Autodesk Fusion 360 part; units mm, degrees
(part 8 of 25)
sketch "Botton Trace" plane through (0, 0, 0) normal (0, 0, 1) x (1, 0, 0)
  arc A0 (82.7578, 33.1788) -> (82.7578, 32.8613) centre (82.7578, 33.0201) ccw
  arc A1 (15.6337, 33.8137) -> (15.6337, 33.4963) centre (15.6337, 33.655) ccw
  arc A2 (82.4468, 33.8137) -> (82.4468, 33.4963) centre (82.4468, 33.655) ccw
  arc A3 (66.04, 33.1788) -> (66.04, 32.8613) centre (66.04, 33.0201) ccw
  arc A4 (81.28, 32.8613) -> (81.28, 33.1788) centre (81.28, 33.0201) ccw
  arc A5 (66.04, 33.4963) -> (66.04, 33.8137) centre (66.04, 33.655) ccw
  arc A6 (0.7747, 33.8137) -> (0.7747, 33.4963) centre (0.7747, 33.655) ccw
  arc A7 (52.818, 33.8137) -> (52.818, 33.4963) centre (52.818, 33.655) ccw
  arc A8 (15.7861, 33.4963) -> (15.7861, 33.8137) centre (15.7861, 33.655) ccw
  arc A9 (71.8947, 32.8613) -> (71.8947, 33.1788) centre (71.8947, 33.0201) ccw
  arc A10 (81.28, 33.8137) -> (81.28, 33.4963) centre (81.28, 33.655) ccw
  arc A11 (35.9156, 33.8137) -> (35.9156, 33.4963) centre (35.9156, 33.655) ccw
  arc A12 (39.1736, 33.4963) -> (39.1736, 33.8137) centre (39.1736, 33.655) ccw
  arc A13 (11.289, 33.8137) -> (11.289, 33.4963) centre (11.289, 33.655) ccw
  arc A14 (52.2859, 33.1788) -> (52.2859, 32.8613) centre (52.2859, 33.0201) ccw
  arc A15 (33.2611, 32.8613) -> (33.2611, 33.1788) centre (33.2611, 33.0201) ccw
  arc A16 (84.2253, 32.8613) -> (84.2253, 33.1788) centre (84.2253, 33.0201) ccw
  arc A17 (17.7419, 33.8137) -> (17.7419, 33.4963) centre (17.7419, 33.655) ccw
  arc A18 (35.3189, 33.1788) -> (35.3189, 32.8613) centre (35.3189, 33.0201) ccw
  arc A19 (31.002, 33.4963) -> (31.002, 33.8137) centre (31.002, 33.655) ccw
  arc A20 (48.6064, 33.1788) -> (48.6064, 32.8613) centre (48.6064, 33.0201) ccw
  arc A21 (17.7419, 33.1788) -> (17.7419, 32.8613) centre (17.7419, 33.0201) ccw
  arc A22 (49.3141, 32.8613) -> (49.3141, 33.1788) centre (49.3141, 33.0201) ccw
  arc A23 (54.9021, 32.8613) -> (54.9021, 33.1788) centre (54.9021, 33.0201) ccw
  arc A24 (84.2253, 33.4963) -> (84.2253, 33.8137) centre (84.2253, 33.655) ccw
  arc A25 (28.2956, 34.4487) -> (28.2956, 34.1313) centre (28.2956, 34.29) ccw
  arc A26 (0.7747, 35.0838) -> (0.7747, 34.7663) centre (0.7747, 34.925) ccw
  line L0 (61.7097, 34.29) -> (62.7503, 34.29)
  arc A27 (84.2253, 34.1313) -> (84.2253, 34.4487) centre (84.2253, 34.29) ccw
  arc A28 (72.517, 34.1313) -> (72.517, 34.4487) centre (72.517, 34.29) ccw
  arc A29 (61.7097, 34.4487) -> (61.7097, 34.1313) centre (61.7097, 34.29) ccw
  arc A30 (17.7419, 34.4487) -> (17.7419, 34.1313) centre (17.7419, 34.29) ccw
  arc A31 (79.7179, 34.4487) -> (79.7179, 34.1313) centre (79.7179, 34.29) ccw
  arc A32 (25.0444, 34.1313) -> (25.0444, 34.4487) centre (25.0444, 34.29) ccw
  arc A33 (56.974, 35.0838) -> (56.974, 34.7663) centre (56.974, 34.925) ccw
  arc A34 (57.1337, 34.4487) -> (57.1337, 34.1313) centre (57.1337, 34.29) ccw
  arc A35 (12.6332, 34.7663) -> (12.6332, 35.0838) centre (12.6332, 34.925) ccw
  arc A36 (60.2103, 34.1313) -> (60.2103, 34.4487) centre (60.2103, 34.29) ccw
  arc A37 (15.613, 34.4487) -> (15.613, 34.1313) centre (15.613, 34.29) ccw
  arc A38 (30.367, 34.1313) -> (30.367, 34.4487) centre (30.367, 34.29) ccw
  arc A39 (54.6263, 34.1313) -> (54.6263, 34.4487) centre (54.6263, 34.29) ccw
  arc A40 (39.8086, 34.1313) -> (39.8086, 34.4487) centre (39.8086, 34.29) ccw
  arc A41 (49.9686, 34.1313) -> (49.9686, 34.4487) centre (49.9686, 34.29) ccw
  arc A42 (35.9156, 34.4487) -> (35.9156, 34.1313) centre (35.9156, 34.29) ccw
  arc A43 (1.0423, 34.7663) -> (1.0423, 35.0838) centre (1.0423, 34.925) ccw
  arc A44 (53.453, 34.4487) -> (53.453, 34.1313) centre (53.453, 34.29) ccw
  arc A45 (62.7503, 34.1313) -> (62.7503, 34.4487) centre (62.7503, 34.29) ccw
  arc A46 (39.0236, 32.8613) -> (39.0236, 33.1788) centre (39.0236, 33.0201) ccw
  arc A47 (81.28, 33.1788) -> (81.28, 32.8613) centre (81.28, 33.0201) ccw
  arc A48 (79.7179, 35.0838) -> (79.7179, 34.7663) centre (79.7179, 34.925) ccw
  arc A49 (41.4714, 34.4487) -> (41.4714, 34.1313) centre (41.4714, 34.29) ccw
  arc A50 (72.517, 34.7663) -> (72.517, 35.0838) centre (72.517, 34.925) ccw
  arc A51 (54.088, 35.0838) -> (54.088, 34.7663) centre (54.088, 34.925) ccw
  arc A52 (10.654, 34.4487) -> (10.654, 34.1313) centre (10.654, 34.29) ccw
  arc A53 (84.2253, 34.7663) -> (84.2253, 35.0838) centre (84.2253, 34.925) ccw
  arc A54 (12.3063, 33.4963) -> (12.3063, 33.8137) centre (12.3063, 33.655) ccw
  arc A55 (15.7861, 34.7663) -> (15.7861, 35.0838) centre (15.7861, 34.925) ccw
  arc A56 (66.04, 32.8613) -> (66.04, 33.1788) centre (66.04, 33.0201) ccw
  arc A57 (25.0444, 33.4963) -> (25.0444, 33.8137) centre (25.0444, 33.655) ccw
  arc A58 (15.7861, 34.1313) -> (15.7861, 34.4487) centre (15.7861, 34.29) ccw
  arc A59 (25.6411, 32.8613) -> (25.6411, 33.1788) centre (25.6411, 33.0201) ccw
  arc A60 (56.8579, 33.1788) -> (56.8579, 32.8613) centre (56.8579, 33.0201) ccw
  arc A61 (0.9017, 34.1313) -> (0.9017, 34.4487) centre (0.9017, 34.29) ccw
  arc A62 (29.5021, 36.6713) -> (29.5021, 36.9887) centre (29.5021, 36.83) ccw
  arc A63 (72.214, 36.3537) -> (72.214, 36.0363) centre (72.214, 36.195) ccw
  arc A64 (4.5252, 35.7188) -> (4.5252, 35.4013) centre (4.5252, 35.5601) ccw
  arc A65 (15.7861, 35.4013) -> (15.7861, 35.7188) centre (15.7861, 35.5601) ccw
  arc A66 (6.6508, 35.4013) -> (6.6508, 35.7188) centre (6.6508, 35.5601) ccw
  arc A67 (72.517, 35.4013) -> (72.517, 35.7188) centre (72.517, 35.5601) ccw
  arc A68 (17.7419, 35.7188) -> (17.7419, 35.4013) centre (17.7419, 35.5601) ccw
  arc A69 (25.6411, 35.4013) -> (25.6411, 35.7188) centre (25.6411, 35.5601) ccw
  arc A70 (72.517, 36.0363) -> (72.517, 36.3537) centre (72.517, 36.195) ccw
  arc A71 (25.0444, 34.7663) -> (25.0444, 35.0838) centre (25.0444, 34.925) ccw
  arc A72 (51.322, 34.7663) -> (51.322, 35.0838) centre (51.322, 34.925) ccw
  arc A73 (27.6989, 36.9887) -> (27.6989, 36.6713) centre (27.6989, 36.83) ccw
  arc A74 (17.7419, 35.0838) -> (17.7419, 34.7663) centre (17.7419, 34.925) ccw
  arc A75 (29.732, 34.7663) -> (29.732, 35.0838) centre (29.732, 34.925) ccw
  arc A76 (64.2497, 34.4487) -> (64.2497, 34.1313) centre (64.2497, 34.29) ccw
  arc A77 (52.592, 36.0363) -> (52.592, 36.3537) centre (52.592, 36.195) ccw
  arc A78 (0.7747, 35.7188) -> (0.7747, 35.4013) centre (0.7747, 35.5601) ccw
  arc A79 (15.3068, 35.0838) -> (15.3068, 34.7663) centre (15.3068, 34.925) ccw
  arc A80 (35.9156, 35.0838) -> (35.9156, 34.7663) centre (35.9156, 34.925) ccw
  arc A81 (11.0836, 36.6713) -> (11.0836, 36.9887) centre (11.0836, 36.83) ccw
  arc A82 (84.2253, 35.4013) -> (84.2253, 35.7188) centre (84.2253, 35.5601) ccw
  arc A83 (14.3164, 36.9887) -> (14.3164, 36.6713) centre (14.3164, 36.83) ccw
  arc A84 (29.5021, 35.4013) -> (29.5021, 35.7188) centre (29.5021, 35.5601) ccw
  arc A85 (1.5708, 35.4013) -> (1.5708, 35.7188) centre (1.5708, 35.5601) ccw
  arc A86 (28.2956, 35.0838) -> (28.2956, 34.7663) centre (28.2956, 34.925) ccw
  arc A87 (29.5021, 36.0363) -> (29.5021, 36.3537) centre (29.5021, 36.195) ccw
  arc A88 (15.7861, 36.0363) -> (15.7861, 36.3537) centre (15.7861, 36.195) ccw
  arc A89 (10.1337, 35.0838) -> (10.1337, 34.7663) centre (10.1337, 34.925) ccw
  arc A90 (54.786, 34.7663) -> (54.786, 35.0838) centre (54.786, 34.925) ccw
  arc A91 (12.327, 34.1313) -> (12.327, 34.4487) centre (12.327, 34.29) ccw
  arc A92 (12.3536, 35.4013) -> (12.3536, 35.7188) centre (12.3536, 35.5601) ccw
  arc A93 (25.6921, 36.0363) -> (25.6921, 36.3537) centre (25.6921, 36.195) ccw
  arc A94 (17.7419, 36.3537) -> (17.7419, 36.0363) centre (17.7419, 36.195) ccw
  arc A95 (79.7179, 35.7188) -> (79.7179, 35.4013) centre (79.7179, 35.5601) ccw
  arc A96 (27.6989, 35.7188) -> (27.6989, 35.4013) centre (27.6989, 35.5601) ccw
  arc A97 (25.6411, 36.6713) -> (25.6411, 36.9887) centre (25.6411, 36.83) ccw
  arc A98 (15.113, 35.7188) -> (15.113, 35.4013) centre (15.113, 35.5601) ccw
  arc A99 (0.7747, 34.4487) -> (0.7747, 34.1313) centre (0.7747, 34.29) ccw
  arc A100 (27.6479, 36.3537) -> (27.6479, 36.0363) centre (27.6479, 36.195) ccw
  arc A101 (33.2611, 36.6713) -> (33.2611, 36.9887) centre (33.2611, 36.83) ccw
  arc A102 (0.7747, 36.3537) -> (0.7747, 36.0363) centre (0.7747, 36.195) ccw
  arc A103 (31.4579, 36.3537) -> (31.4579, 36.0363) centre (31.4579, 36.195) ccw
  arc A104 (84.2253, 36.0363) -> (84.2253, 36.3537) centre (84.2253, 36.195) ccw
  arc A105 (31.4579, 36.9887) -> (31.4579, 36.6713) centre (31.4579, 36.83) ccw
  arc A106 (35.3189, 36.9887) -> (35.3189, 36.6713) centre (35.3189, 36.83) ccw
  arc A107 (17.7419, 36.9887) -> (17.7419, 36.6713) centre (17.7419, 36.83) ccw
  arc A108 (51.6314, 36.9887) -> (51.6314, 36.6713) centre (51.6314, 36.83) ccw
  arc A109 (51.957, 35.4013) -> (51.957, 35.7188) centre (51.957, 35.5601) ccw
  arc A110 (79.7179, 36.3537) -> (79.7179, 36.0363) centre (79.7179, 36.195) ccw
  arc A111 (31.863, 35.7188) -> (31.863, 35.4013) centre (31.863, 35.5601) ccw
  arc A112 (9.6052, 35.7188) -> (9.6052, 35.4013) centre (9.6052, 35.5601) ccw
  arc A113 (72.214, 37.6238) -> (72.214, 37.3063) centre (72.214, 37.4651) ccw
  arc A114 (20.32, 37.9413) -> (20.32, 38.2587) centre (20.32, 38.1) ccw
  arc A115 (39.8086, 36.6713) -> (39.8086, 36.9887) centre (39.8086, 36.83) ccw
  arc A116 (33.2611, 35.4013) -> (33.2611, 35.7188) centre (33.2611, 35.5601) ccw
  arc A117 (0.7747, 36.9887) -> (0.7747, 36.6713) centre (0.7747, 36.83) ccw
  arc A118 (31.4579, 37.6238) -> (31.4579, 37.3063) centre (31.4579, 37.4651) ccw
  arc A119 (84.2253, 36.6713) -> (84.2253, 36.9887) centre (84.2253, 36.83) ccw
  arc A120 (18.6006, 37.3063) -> (18.6006, 37.6238) centre (18.6006, 37.4651) ccw
  arc A121 (79.7179, 36.9887) -> (79.7179, 36.6713) centre (79.7179, 36.83) ccw
  arc A122 (17.7419, 37.6238) -> (17.7419, 37.3063) centre (17.7419, 37.4651) ccw
  arc A123 (25.0444, 37.3063) -> (25.0444, 37.6238) centre (25.0444, 37.4651) ccw
  arc A124 (0.7747, 38.2587) -> (0.7747, 37.9413) centre (0.7747, 38.1) ccw
  arc A125 (3.4636, 37.9413) -> (3.4636, 38.2587) centre (3.4636, 38.1) ccw
  arc A126 (28.2956, 37.6238) -> (28.2956, 37.3063) centre (28.2956, 37.4651) ccw
  arc A127 (13.6814, 37.6238) -> (13.6814, 37.3063) centre (13.6814, 37.4651) ccw
  arc A128 (39.1736, 37.3063) -> (39.1736, 37.6238) centre (39.1736, 37.4651) ccw
  arc A129 (15.7861, 36.6713) -> (15.7861, 36.9887) centre (15.7861, 36.83) ccw
  arc A130 (17.7419, 38.2587) -> (17.7419, 37.9413) centre (17.7419, 38.1) ccw
  arc A131 (72.517, 36.6713) -> (72.517, 36.9887) centre (72.517, 36.83) ccw
  arc A132 (20.32, 37.6238) -> (20.32, 37.3063) centre (20.32, 37.4651) ccw
  arc A133 (35.3189, 35.7188) -> (35.3189, 35.4013) centre (35.3189, 35.5601) ccw
  arc A134 (49.9686, 36.6713) -> (49.9686, 36.9887) centre (49.9686, 36.83) ccw
  arc A135 (4.0986, 37.3063) -> (4.0986, 37.6238) centre (4.0986, 37.4651) ccw
  arc A136 (22.0394, 37.6238) -> (22.0394, 37.3063) centre (22.0394, 37.4651) ccw
  arc A137 (11.7186, 36.0363) -> (11.7186, 36.3537) centre (11.7186, 36.195) ccw
  arc A138 (20.32, 37.3063) -> (20.32, 37.6238) centre (20.32, 37.4651) ccw
  arc A139 (20.32, 38.2587) -> (20.32, 37.9413) centre (20.32, 38.1) ccw
  arc A140 (15.7861, 37.9413) -> (15.7861, 38.2587) centre (15.7861, 38.1) ccw
  arc A141 (72.3737, 36.9887) -> (72.3737, 36.6713) centre (72.3737, 36.83) ccw
  arc A142 (41.4714, 36.9887) -> (41.4714, 36.6713) centre (41.4714, 36.83) ccw
  arc A143 (15.7861, 37.3063) -> (15.7861, 37.6238) centre (15.7861, 37.4651) ccw
  arc A144 (53.227, 36.6713) -> (53.227, 36.9887) centre (53.227, 36.83) ccw
  arc A145 (54.723, 35.7188) -> (54.723, 35.4013) centre (54.723, 35.5601) ccw
  arc A146 (14.9442, 36.3537) -> (14.9442, 36.0363) centre (14.9442, 36.195) ccw
  arc A147 (13.0464, 38.2587) -> (13.0464, 37.9413) centre (13.0464, 38.1) ccw
  arc A148 (25.0444, 37.9413) -> (25.0444, 38.2587) centre (25.0444, 38.1) ccw
  arc A149 (29.5021, 37.9413) -> (29.5021, 38.2587) centre (29.5021, 38.1) ccw
  arc A150 (0.7747, 37.6238) -> (0.7747, 37.3063) centre (0.7747, 37.4651) ccw
  arc A151 (49.3336, 38.5763) -> (49.3336, 38.8937) centre (49.3336, 38.735) ccw
  arc A152 (84.2253, 38.5763) -> (84.2253, 38.8937) centre (84.2253, 38.735) ccw
  arc A153 (0.7747, 39.5288) -> (0.7747, 39.2113) centre (0.7747, 39.37) ccw
  arc A154 (72.517, 38.5763) -> (72.517, 38.8937) centre (72.517, 38.735) ccw
  arc A155 (2.8286, 38.5763) -> (2.8286, 38.8937) centre (2.8286, 38.735) ccw
  arc A156 (18.6006, 38.5763) -> (18.6006, 38.8937) centre (18.6006, 38.735) ccw
  arc A157 (79.7179, 38.2587) -> (79.7179, 37.9413) centre (79.7179, 38.1) ccw
  arc A158 (15.7861, 38.5763) -> (15.7861, 38.8937) centre (15.7861, 38.735) ccw
  arc A159 (12.4114, 38.8937) -> (12.4114, 38.5763) centre (12.4114, 38.735) ccw
  arc A160 (2.1936, 39.2113) -> (2.1936, 39.5288) centre (2.1936, 39.37) ccw
  arc A161 (37.578, 37.6238) -> (37.578, 37.3063) centre (37.578, 37.4651) ccw
  arc A162 (49.3336, 37.3063) -> (49.3336, 37.6238) centre (49.3336, 37.4651) ccw
  arc A163 (17.7419, 38.8937) -> (17.7419, 38.5763) centre (17.7419, 38.735) ccw
  arc A164 (21.7972, 39.5288) -> (21.7972, 39.2113) centre (21.7972, 39.37) ccw
  arc A165 (28.2956, 38.8937) -> (28.2956, 38.5763) centre (28.2956, 38.735) ccw
  arc A166 (42.2564, 38.2587) -> (42.2564, 37.9413) centre (42.2564, 38.1) ccw
  arc A167 (38.213, 38.2587) -> (38.213, 37.9413) centre (38.213, 38.1) ccw
  arc A168 (39.1541, 37.9413) -> (39.1541, 38.2587) centre (39.1541, 38.1) ccw
  arc A169 (28.2956, 38.2587) -> (28.2956, 37.9413) centre (28.2956, 38.1) ccw
  arc A170 (27.6989, 39.5288) -> (27.6989, 39.2113) centre (27.6989, 39.37) ccw
  arc A171 (18.8428, 39.2113) -> (18.8428, 39.5288) centre (18.8428, 39.37) ccw
  arc A172 (84.2253, 37.3063) -> (84.2253, 37.6238) centre (84.2253, 37.4651) ccw
  arc A173 (53.862, 37.3063) -> (53.862, 37.6238) centre (53.862, 37.4651) ccw
  arc A174 (32.6644, 37.3063) -> (32.6644, 37.6238) centre (32.6644, 37.4651) ccw
  arc A175 (33.2611, 39.2113) -> (33.2611, 39.5288) centre (33.2611, 39.37) ccw
  arc A176 (22.0394, 38.8937) -> (22.0394, 38.5763) centre (22.0394, 38.735) ccw
  arc A177 (38.848, 38.8937) -> (38.848, 38.5763) centre (38.848, 38.735) ccw
  arc A178 (29.5021, 37.3063) -> (29.5021, 37.6238) centre (29.5021, 37.4651) ccw
  arc A179 (32.6644, 37.9413) -> (32.6644, 38.2587) centre (32.6644, 38.1) ccw
  arc A180 (84.2253, 37.9413) -> (84.2253, 38.2587) centre (84.2253, 38.1) ccw
  arc A181 (42.8914, 38.8937) -> (42.8914, 38.5763) centre (42.8914, 38.735) ccw
  arc A182 (25.0444, 38.5763) -> (25.0444, 38.8937) centre (25.0444, 38.735) ccw
  arc A183 (79.7179, 38.8937) -> (79.7179, 38.5763) centre (79.7179, 38.735) ccw
  arc A184 (25.6411, 39.2113) -> (25.6411, 39.5288) centre (25.6411, 39.37) ccw
  arc A185 (42.1064, 37.6238) -> (42.1064, 37.3063) centre (42.1064, 37.4651) ccw
  arc A186 (79.7179, 37.6238) -> (79.7179, 37.3063) centre (79.7179, 37.4651) ccw
  arc A187 (72.214, 38.8937) -> (72.214, 38.5763) centre (72.214, 38.735) ccw
  arc A188 (52.2664, 37.6238) -> (52.2664, 37.3063) centre (52.2664, 37.4651) ccw
  arc A189 (29.5021, 38.5763) -> (29.5021, 38.8937) centre (29.5021, 38.735) ccw
  arc A190 (72.517, 37.3063) -> (72.517, 37.6238) centre (72.517, 37.4651) ccw
  arc A191 (31.4579, 38.8937) -> (31.4579, 38.5763) centre (31.4579, 38.735) ccw
  arc A192 (39.1736, 38.5763) -> (39.1736, 38.8937) centre (39.1736, 38.735) ccw
  arc A193 (18.3143, 39.8463) -> (18.3143, 40.1638) centre (18.3143, 40.0051) ccw
  arc A194 (32.6644, 38.5763) -> (32.6644, 38.8937) centre (32.6644, 38.735) ccw
  arc A195 (40.9286, 39.8463) -> (40.9286, 40.1638) centre (40.9286, 40.0051) ccw
  arc A196 (5.4264, 39.5288) -> (5.4264, 39.2113) centre (5.4264, 39.37) ccw
  arc A197 (49.3141, 37.9413) -> (49.3141, 38.2587) centre (49.3141, 38.1) ccw
  arc A198 (27.5014, 40.7987) -> (27.5014, 40.4813) centre (27.5014, 40.64) ccw
  arc A199 (72.517, 39.2113) -> (72.517, 39.5288) centre (72.517, 39.37) ccw
  arc A200 (17.7419, 39.5288) -> (17.7419, 39.2113) centre (17.7419, 39.37) ccw
  arc A201 (31.4579, 40.1638) -> (31.4579, 39.8463) centre (31.4579, 40.0051) ccw
  arc A202 (4.5252, 40.7987) -> (4.5252, 40.4813) centre (4.5252, 40.64) ccw
  arc A203 (29.5021, 40.4813) -> (29.5021, 40.7987) centre (29.5021, 40.64) ccw
  arc A204 (35.3189, 39.5288) -> (35.3189, 39.2113) centre (35.3189, 39.37) ccw
  arc A205 (84.2253, 39.2113) -> (84.2253, 39.5288) centre (84.2253, 39.37) ccw
  arc A206 (39.8086, 39.2113) -> (39.8086, 39.5288) centre (39.8086, 39.37) ccw
  arc A207 (9.6052, 40.7987) -> (9.6052, 40.4813) centre (9.6052, 40.64) ccw
  arc A208 (31.4579, 40.7987) -> (31.4579, 40.4813) centre (31.4579, 40.64) ccw
  arc A209 (52.2859, 38.2587) -> (52.2859, 37.9413) centre (52.2859, 38.1) ccw
  arc A210 (72.517, 37.9413) -> (72.517, 38.2587) centre (72.517, 38.1) ccw
  arc A211 (17.7419, 40.1638) -> (17.7419, 39.8463) centre (17.7419, 40.0051) ccw
  arc A212 (26.148, 40.1638) -> (26.148, 39.8463) centre (26.148, 40.0051) ccw
  arc A213 (37.987, 40.4813) -> (37.987, 40.7987) centre (37.987, 40.64) ccw
  arc A214 (49.9686, 39.2113) -> (49.9686, 39.5288) centre (49.9686, 39.37) ccw
  arc A215 (4.7914, 40.1638) -> (4.7914, 39.8463) centre (4.7914, 40.0051) ccw
  arc A216 (37.352, 39.8463) -> (37.352, 40.1638) centre (37.352, 40.0051) ccw
  arc A217 (31.4579, 38.2587) -> (31.4579, 37.9413) centre (31.4579, 38.1) ccw
  arc A218 (79.7179, 39.5288) -> (79.7179, 39.2113) centre (79.7179, 39.37) ccw
  arc A219 (1.905, 39.8463) -> (1.905, 40.1638) centre (1.905, 40.0051) ccw
  arc A220 (0.7747, 40.1638) -> (0.7747, 39.8463) centre (0.7747, 40.0051) ccw
  arc A221 (72.214, 40.1638) -> (72.214, 39.8463) centre (72.214, 40.0051) ccw
  arc A222 (15.7861, 39.2113) -> (15.7861, 39.5288) centre (15.7861, 39.37) ccw
  arc A223 (18.1737, 40.4813) -> (18.1737, 40.7987) centre (18.1737, 40.64) ccw
  arc A224 (35.9986, 40.4813) -> (35.9986, 40.7987) centre (35.9986, 40.64) ccw
  arc A225 (39.483, 39.5288) -> (39.483, 39.2113) centre (39.483, 39.37) ccw
  arc A226 (0.7747, 38.8937) -> (0.7747, 38.5763) centre (0.7747, 38.735) ccw
  arc A227 (17.7419, 40.7987) -> (17.7419, 40.4813) centre (17.7419, 40.64) ccw
  arc A228 (29.5021, 39.2113) -> (29.5021, 39.5288) centre (29.5021, 39.37) ccw
  arc A229 (72.3737, 39.5288) -> (72.3737, 39.2113) centre (72.3737, 39.37) ccw
  arc A230 (50.5114, 40.1638) -> (50.5114, 39.8463) centre (50.5114, 40.0051) ccw
  arc A231 (37.6614, 40.7987) -> (37.6614, 40.4813) centre (37.6614, 40.64) ccw
  arc A232 (36.717, 39.2113) -> (36.717, 39.5288) centre (36.717, 39.37) ccw
  arc A233 (43.5264, 39.5288) -> (43.5264, 39.2113) centre (43.5264, 39.37) ccw
  arc A234 (42.1986, 41.1163) -> (42.1986, 41.4337) centre (42.1986, 41.275) ccw
  arc A235 (66.04, 41.4337) -> (66.04, 41.1163) centre (66.04, 41.275) ccw
  arc A236 (29.5021, 39.8463) -> (29.5021, 40.1638) centre (29.5021, 40.0051) ccw
  arc A237 (18.8428, 41.7513) -> (18.8428, 42.0688) centre (18.8428, 41.9101) ccw
  arc A238 (79.7179, 40.1638) -> (79.7179, 39.8463) centre (79.7179, 40.0051) ccw
  arc A239 (0.7747, 41.4337) -> (0.7747, 41.1163) centre (0.7747, 41.275) ccw
  arc A240 (38.2964, 41.4337) -> (38.2964, 41.1163) centre (38.2964, 41.275) ccw
  arc A241 (72.517, 39.8463) -> (72.517, 40.1638) centre (72.517, 40.0051) ccw
  arc A242 (60.2103, 40.4813) -> (60.2103, 40.7987) centre (60.2103, 40.64) ccw
  arc A243 (62.7503, 40.4813) -> (62.7503, 40.7987) centre (62.7503, 40.64) ccw
  arc A244 (51.6314, 40.7987) -> (51.6314, 40.4813) centre (51.6314, 40.64) ccw
  arc A245 (51.322, 39.8463) -> (51.322, 40.1638) centre (51.322, 40.0051) ccw
  arc A246 (31.4579, 39.5288) -> (31.4579, 39.2113) centre (31.4579, 39.37) ccw
  arc A247 (64.2497, 40.7987) -> (64.2497, 40.4813) centre (64.2497, 40.64) ccw
  arc A248 (72.517, 41.1163) -> (72.517, 41.4337) centre (72.517, 41.275) ccw
  arc A249 (5.0537, 41.4337) -> (5.0537, 41.1163) centre (5.0537, 41.275) ccw
  arc A250 (79.7179, 40.7987) -> (79.7179, 40.4813) centre (79.7179, 40.64) ccw
  arc A251 (42.1064, 41.4337) -> (42.1064, 41.1163) centre (42.1064, 41.275) ccw
  arc A252 (28.1364, 41.4337) -> (28.1364, 41.1163) centre (28.1364, 41.275) ccw
  arc A253 (59.1697, 40.7987) -> (59.1697, 40.4813) centre (59.1697, 40.64) ccw
  arc A254 (6.6508, 40.4813) -> (6.6508, 40.7987) centre (6.6508, 40.64) ccw
  arc A255 (72.517, 40.4813) -> (72.517, 40.7987) centre (72.517, 40.64) ccw
  arc A256 (56.9091, 41.1163) -> (56.9091, 41.4337) centre (56.9091, 41.275) ccw
  arc A257 (6.1223, 41.1163) -> (6.1223, 41.4337) centre (6.1223, 41.275) ccw
  arc A258 (15.7861, 40.4813) -> (15.7861, 40.7987) centre (15.7861, 40.64) ccw
  arc A259 (66.04, 41.1163) -> (66.04, 41.4337) centre (66.04, 41.275) ccw
  arc A260 (15.7861, 41.7513) -> (15.7861, 42.0688) centre (15.7861, 41.9101) ccw
  arc A261 (10.908, 41.4337) -> (10.908, 41.1163) centre (10.908, 41.275) ccw
  arc A262 (61.7097, 40.7987) -> (61.7097, 40.4813) centre (61.7097, 40.64) ccw
  arc A263 (15.7861, 41.1163) -> (15.7861, 41.4337) centre (15.7861, 41.275) ccw
  arc A264 (1.5708, 40.4813) -> (1.5708, 40.7987) centre (1.5708, 40.64) ccw
  arc A265 (1.0423, 41.1163) -> (1.0423, 41.4337) centre (1.0423, 41.275) ccw
  arc A266 (84.2253, 39.8463) -> (84.2253, 40.1638) centre (84.2253, 40.0051) ccw
  arc A267 (41.5636, 40.4813) -> (41.5636, 40.7987) centre (41.5636, 40.64) ccw
  arc A268 (5.1943, 42.0688) -> (5.1943, 41.7513) centre (5.1943, 41.9101) ccw
  arc A269 (0.7747, 40.7987) -> (0.7747, 40.4813) centre (0.7747, 40.64) ccw
  arc A270 (15.7861, 39.8463) -> (15.7861, 40.1638) centre (15.7861, 40.0051) ccw
  arc A271 (11.543, 42.0688) -> (11.543, 41.7513) centre (11.543, 41.9101) ccw
  arc A272 (84.2253, 40.4813) -> (84.2253, 40.7987) centre (84.2253, 40.64) ccw
  arc A273 (17.7419, 41.4337) -> (17.7419, 41.1163) centre (17.7419, 41.275) ccw
  arc A274 (35.3636, 41.1163) -> (35.3636, 41.4337) centre (35.3636, 41.275) ccw
  arc A275 (40.118, 40.1638) -> (40.118, 39.8463) centre (40.118, 40.0051) ccw
  arc A276 (41.4714, 40.7987) -> (41.4714, 40.4813) centre (41.4714, 40.64) ccw
  arc A277 (18.3143, 41.1163) -> (18.3143, 41.4337) centre (18.3143, 41.275) ccw
  arc A278 (66.04, 42.7037) -> (66.04, 42.3863) centre (66.04, 42.545) ccw
  arc A279 (81.28, 42.3863) -> (81.28, 42.7037) centre (81.28, 42.545) ccw
  arc A280 (39.1736, 42.3863) -> (39.1736, 42.7037) centre (39.1736, 42.545) ccw
  arc A281 (38.2964, 42.7037) -> (38.2964, 42.3863) centre (38.2964, 42.545) ccw
  arc A282 (28.1559, 42.0688) -> (28.1559, 41.7513) centre (28.1559, 41.9101) ccw
  arc A283 (31.4579, 41.4337) -> (31.4579, 41.1163) centre (31.4579, 41.275) ccw
  arc A284 (32.498, 42.7037) -> (32.498, 42.3863) centre (32.498, 42.545) ccw
  arc A285 (42.658, 42.7037) -> (42.658, 42.3863) centre (42.658, 42.545) ccw
  arc A286 (25.1841, 41.7513) -> (25.1841, 42.0688) centre (25.1841, 41.9101) ccw
  arc A287 (72.517, 41.7513) -> (72.517, 42.0688) centre (72.517, 41.9101) ccw
  arc A288 (57.6703, 40.4813) -> (57.6703, 40.7987) centre (57.6703, 40.64) ccw
  arc A289 (29.732, 42.3863) -> (29.732, 42.7037) centre (29.732, 42.545) ccw
  arc A290 (67.2068, 41.4337) -> (67.2068, 41.1163) centre (67.2068, 41.275) ccw
  arc A291 (0.9017, 41.7513) -> (0.9017, 42.0688) centre (0.9017, 41.9101) ccw
  arc A292 (29.5021, 41.7513) -> (29.5021, 42.0688) centre (29.5021, 41.9101) ccw
  arc A293 (79.7179, 42.0688) -> (79.7179, 41.7513) centre (79.7179, 41.9101) ccw
  arc A294 (31.863, 42.0688) -> (31.863, 41.7513) centre (31.863, 41.9101) ccw
  arc A295 (84.2253, 41.7513) -> (84.2253, 42.0688) centre (84.2253, 41.9101) ccw
  arc A296 (5.0537, 42.7037) -> (5.0537, 42.3863) centre (5.0537, 42.545) ccw
  arc A297 (13.3018, 42.3863) -> (13.3018, 42.7037) centre (13.3018, 42.545) ccw
  arc A298 (66.04, 42.3863) -> (66.04, 42.7037) centre (66.04, 42.545) ccw
  arc A299 (42.1259, 42.0688) -> (42.1259, 41.7513) centre (42.1259, 41.9101) ccw
  arc A300 (17.7419, 42.7037) -> (17.7419, 42.3863) centre (17.7419, 42.545) ccw
  arc A301 (0.7747, 42.7037) -> (0.7747, 42.3863) centre (0.7747, 42.545) ccw
  arc A302 (79.7179, 41.4337) -> (79.7179, 41.1163) centre (79.7179, 41.275) ccw
  arc A303 (52.2664, 41.4337) -> (52.2664, 41.1163) centre (52.2664, 41.275) ccw
  arc A304 (0.7747, 42.0688) -> (0.7747, 41.7513) centre (0.7747, 41.9101) ccw
  arc A305 (35.3441, 41.7513) -> (35.3441, 42.0688) centre (35.3441, 41.9101) ccw
  arc A306 (81.28, 42.7037) -> (81.28, 42.3863) centre (81.28, 42.545) ccw
  arc A307 (21.7972, 42.0688) -> (21.7972, 41.7513) centre (21.7972, 41.9101) ccw
  arc A308 (15.7861, 42.3863) -> (15.7861, 42.7037) centre (15.7861, 42.545) ccw
  arc A309 (1.0423, 42.3863) -> (1.0423, 42.7037) centre (1.0423, 42.545) ccw
  arc A310 (67.5513, 42.7037) -> (67.5513, 42.3863) centre (67.5513, 42.545) ccw
  arc A311 (5.9817, 41.7513) -> (5.9817, 42.0688) centre (5.9817, 41.9101) ccw
  arc A312 (66.04, 41.7513) -> (66.04, 42.0688) centre (66.04, 41.9101) ccw
  arc A313 (49.3336, 42.3863) -> (49.3336, 42.7037) centre (49.3336, 42.545) ccw
  arc A314 (38.3159, 42.0688) -> (38.3159, 41.7513) centre (38.3159, 41.9101) ccw
  arc A315 (84.2253, 41.1163) -> (84.2253, 41.4337) centre (84.2253, 41.275) ccw
  arc A316 (28.1364, 42.7037) -> (28.1364, 42.3863) centre (28.1364, 42.545) ccw
  arc A317 (52.4164, 42.0688) -> (52.4164, 41.7513) centre (52.4164, 41.9101) ccw
  arc A318 (56.6547, 41.7513) -> (56.6547, 42.0688) centre (56.6547, 41.9101) ccw
  arc A319 (29.5021, 41.1163) -> (29.5021, 41.4337) centre (29.5021, 41.275) ccw
  arc A320 (38.622, 41.1163) -> (38.622, 41.4337) centre (38.622, 41.275) ccw
  arc A321 (72.1491, 42.3863) -> (72.1491, 42.7037) centre (72.1491, 42.545) ccw
  arc A322 (39.1541, 41.7513) -> (39.1541, 42.0688) centre (39.1541, 41.9101) ccw
  arc A323 (12.178, 42.7037) -> (12.178, 42.3863) centre (12.178, 42.545) ccw
  arc A324 (66.04, 43.6563) -> (66.04, 43.9738) centre (66.04, 43.815) ccw
  arc A325 (43.293, 43.3387) -> (43.293, 43.0213) centre (43.293, 43.18) ccw
  arc A326 (17.7419, 43.3387) -> (17.7419, 43.0213) centre (17.7419, 43.18) ccw
  arc A327 (15.4025, 43.3387) -> (15.4025, 43.0213) centre (15.4025, 43.18) ccw
  arc A328 (14.6382, 42.7037) -> (14.6382, 42.3863) centre (14.6382, 42.545) ccw
  arc A329 (15.7861, 43.0213) -> (15.7861, 43.3387) centre (15.7861, 43.18) ccw
  arc A330 (25.2036, 42.3863) -> (25.2036, 42.7037) centre (25.2036, 42.545) ccw
  arc A331 (41.162, 43.6563) -> (41.162, 43.9738) centre (41.162, 43.815) ccw
  arc A332 (81.28, 43.6563) -> (81.28, 43.9738) centre (81.28, 43.815) ccw
  arc A333 (84.2253, 43.0213) -> (84.2253, 43.3387) centre (84.2253, 43.18) ccw
  arc A334 (66.04, 43.9738) -> (66.04, 43.6563) centre (66.04, 43.815) ccw
  arc A335 (27.5014, 43.3387) -> (27.5014, 43.0213) centre (27.5014, 43.18) ccw
  arc A336 (18.1737, 43.0213) -> (18.1737, 43.3387) centre (18.1737, 43.18) ccw
  arc A337 (35.9986, 43.0213) -> (35.9986, 43.3387) centre (35.9986, 43.18) ccw
  arc A338 (31.002, 43.6563) -> (31.002, 43.9738) centre (31.002, 43.815) ccw
  arc A339 (0.7747, 43.3387) -> (0.7747, 43.0213) centre (0.7747, 43.18) ccw
  arc A340 (35.3636, 42.3863) -> (35.3636, 42.7037) centre (35.3636, 42.545) ccw
  arc A341 (81.28, 43.0213) -> (81.28, 43.3387) centre (81.28, 43.18) ccw
  arc A342 (33.133, 43.3387) -> (33.133, 43.0213) centre (33.133, 43.18) ccw
  arc A343 (0.7747, 43.9738) -> (0.7747, 43.6563) centre (0.7747, 43.815) ccw
  arc A344 (49.9686, 43.0213) -> (49.9686, 43.3387) centre (49.9686, 43.18) ccw
  arc A345 (84.2253, 42.3863) -> (84.2253, 42.7037) centre (84.2253, 42.545) ccw
  arc A346 (81.28, 43.3387) -> (81.28, 43.0213) centre (81.28, 43.18) ccw
  arc A347 (1.0423, 43.6563) -> (1.0423, 43.9738) centre (1.0423, 43.815) ccw
  arc A348 (67.5513, 43.9738) -> (67.5513, 43.6563) centre (67.5513, 43.815) ccw
  arc A349 (6.1223, 42.3863) -> (6.1223, 42.7037) centre (6.1223, 42.545) ccw
  arc A350 (39.8086, 43.0213) -> (39.8086, 43.3387) centre (39.8086, 43.18) ccw
  arc A351 (18.3143, 42.3863) -> (18.3143, 42.7037) centre (18.3143, 42.545) ccw
  arc A352 (6.6508, 43.0213) -> (6.6508, 43.3387) centre (6.6508, 43.18) ccw
  arc A353 (4.5252, 43.3387) -> (4.5252, 43.0213) centre (4.5252, 43.18) ccw
  arc A354 (17.7419, 42.0688) -> (17.7419, 41.7513) centre (17.7419, 41.9101) ccw
  arc A355 (49.1836, 41.7513) -> (49.1836, 42.0688) centre (49.1836, 41.9101) ccw
  arc A356 (22.3257, 42.7037) -> (22.3257, 42.3863) centre (22.3257, 42.545) ccw
  arc A357 (17.7419, 43.9738) -> (17.7419, 43.6563) centre (17.7419, 43.815) ccw
  arc A358 (67.5178, 42.0688) -> (67.5178, 41.7513) centre (67.5178, 41.9101) ccw
  arc A359 (82.4468, 42.7037) -> (82.4468, 42.3863) centre (82.4468, 42.545) ccw
  arc A360 (40.118, 43.9738) -> (40.118, 43.6563) centre (40.118, 43.815) ccw
  arc A361 (22.4663, 43.3387) -> (22.4663, 43.0213) centre (22.4663, 43.18) ccw
  arc A362 (71.8947, 43.6563) -> (71.8947, 43.9738) centre (71.8947, 43.815) ccw
  arc A363 (22.3257, 43.9738) -> (22.3257, 43.6563) centre (22.3257, 43.815) ccw
  arc A364 (81.28, 43.9738) -> (81.28, 43.6563) centre (81.28, 43.815) ccw
  arc A365 (66.04, 42.0688) -> (66.04, 41.7513) centre (66.04, 41.9101) ccw
  arc A366 (25.8386, 43.0213) -> (25.8386, 43.3387) centre (25.8386, 43.18) ccw
  arc A367 (15.6337, 43.9738) -> (15.6337, 43.6563) centre (15.6337, 43.815) ccw
  arc A368 (81.28, 45.2437) -> (81.28, 44.9263) centre (81.28, 45.085) ccw
  arc A369 (0.7747, 44.6088) -> (0.7747, 44.2913) centre (0.7747, 44.4501) ccw
  arc A370 (15.762, 43.6563) -> (15.762, 43.9738) centre (15.762, 43.815) ccw
  arc A371 (81.28, 44.9263) -> (81.28, 45.2437) centre (81.28, 45.085) ccw
  arc A372 (21.7972, 44.6088) -> (21.7972, 44.2913) centre (21.7972, 44.4501) ccw
  arc A373 (66.04, 45.2437) -> (66.04, 44.9263) centre (66.04, 45.085) ccw
  arc A374 (17.7173, 44.6088) -> (17.7173, 44.2913) centre (17.7173, 44.4501) ccw
  arc A375 (82.7913, 43.9738) -> (82.7913, 43.6563) centre (82.7913, 43.815) ccw
  arc A376 (41.388, 45.2437) -> (41.388, 44.9263) centre (41.388, 45.085) ccw
  arc A377 (66.04, 44.6088) -> (66.04, 44.2913) centre (66.04, 44.4501) ccw
  arc A378 (1.5708, 43.0213) -> (1.5708, 43.3387) centre (1.5708, 43.18) ccw
  arc A379 (37.6614, 43.3387) -> (37.6614, 43.0213) centre (37.6614, 43.18) ccw
  arc A380 (10.047, 45.5613) -> (10.047, 45.8787) centre (10.047, 45.72) ccw
  arc A381 (6.6508, 45.5613) -> (6.6508, 45.8787) centre (6.6508, 45.72) ccw
  arc A382 (1.5708, 45.5613) -> (1.5708, 45.8787) centre (1.5708, 45.72) ccw
  arc A383 (18.3143, 43.6563) -> (18.3143, 43.9738) centre (18.3143, 43.815) ccw
  arc A384 (6.1223, 43.6563) -> (6.1223, 43.9738) centre (6.1223, 43.815) ccw
  arc A385 (66.04, 43.3387) -> (66.04, 43.0213) centre (66.04, 43.18) ccw
  arc A386 (40.753, 44.6088) -> (40.753, 44.2913) centre (40.753, 44.4501) ccw
  arc A387 (66.04, 44.2913) -> (66.04, 44.6088) centre (66.04, 44.4501) ccw
  arc A388 (23.5113, 45.5613) -> (23.5113, 45.8787) centre (23.5113, 45.72) ccw
  arc A389 (81.28, 44.6088) -> (81.28, 44.2913) centre (81.28, 44.4501) ccw
  arc A390 (41.797, 44.2913) -> (41.797, 44.6088) centre (41.797, 44.4501) ccw
  arc A391 (9.6052, 45.8787) -> (9.6052, 45.5613) centre (9.6052, 45.72) ccw
  arc A392 (67.2068, 45.2437) -> (67.2068, 44.9263) centre (67.2068, 45.085) ccw
  arc A393 (0.9017, 44.2913) -> (0.9017, 44.6088) centre (0.9017, 44.4501) ccw
  arc A394 (71.8947, 44.2913) -> (71.8947, 44.6088) centre (71.8947, 44.4501) ccw
  arc A395 (23.671, 44.9263) -> (23.671, 45.2437) centre (23.671, 45.085) ccw
  arc A396 (54.5937, 44.6088) -> (54.5937, 44.2913) centre (54.5937, 44.4501) ccw
  arc A397 (84.2253, 43.6563) -> (84.2253, 43.9738) centre (84.2253, 43.815) ccw
  arc A398 (5.0537, 43.9738) -> (5.0537, 43.6563) centre (5.0537, 43.815) ccw
  arc A399 (30.367, 43.0213) -> (30.367, 43.3387) centre (30.367, 43.18) ccw
  arc A400 (56.6547, 44.2913) -> (56.6547, 44.6088) centre (56.6547, 44.4501) ccw
  arc A401 (6.1223, 44.9263) -> (6.1223, 45.2437) centre (6.1223, 45.085) ccw
  arc A402 (1.0423, 44.9263) -> (1.0423, 45.2437) centre (1.0423, 45.085) ccw
  arc A403 (82.7578, 43.3387) -> (82.7578, 43.0213) centre (82.7578, 43.18) ccw
  arc A404 (82.7913, 45.2437) -> (82.7913, 44.9263) centre (82.7913, 45.085) ccw
  arc A405 (5.1943, 44.6088) -> (5.1943, 44.2913) centre (5.1943, 44.4501) ccw
  arc A406 (18.8428, 44.2913) -> (18.8428, 44.6088) centre (18.8428, 44.4501) ccw
  arc A407 (84.2253, 44.9263) -> (84.2253, 45.2437) centre (84.2253, 45.085) ccw
  arc A408 (71.8947, 43.0213) -> (71.8947, 43.3387) centre (71.8947, 43.18) ccw
  arc A409 (4.5252, 45.8787) -> (4.5252, 45.5613) centre (4.5252, 45.72) ccw
  arc A410 (67.5178, 44.6088) -> (67.5178, 44.2913) centre (67.5178, 44.4501) ccw
  arc A411 (31.637, 44.2913) -> (31.637, 44.6088) centre (31.637, 44.4501) ccw
  arc A412 (42.432, 44.9263) -> (42.432, 45.2437) centre (42.432, 45.085) ccw
  arc A413 (56.9091, 44.9263) -> (56.9091, 45.2437) centre (56.9091, 45.085) ccw
  arc A414 (66.04, 44.9263) -> (66.04, 45.2437) centre (66.04, 45.085) ccw
  arc A415 (5.0537, 45.2437) -> (5.0537, 44.9263) centre (5.0537, 45.085) ccw
  arc A416 (79.4897, 47.1487) -> (79.4897, 46.8313) centre (79.4897, 46.99) ccw
  arc A417 (54.434, 45.2437) -> (54.434, 44.9263) centre (54.434, 45.085) ccw
  arc A418 (71.8947, 45.5613) -> (71.8947, 45.8787) centre (71.8947, 45.72) ccw
  arc A419 (15.7603, 46.8313) -> (15.7603, 47.1487) centre (15.7603, 46.99) ccw
  arc A420 (84.2253, 46.8313) -> (84.2253, 47.1487) centre (84.2253, 46.99) ccw
  arc A421 (17.2597, 47.1487) -> (17.2597, 46.8313) centre (17.2597, 46.99) ccw
  arc A422 (9.9191, 47.4663) -> (9.9191, 47.7837) centre (9.9191, 47.625) ccw
  arc A423 (61.073, 47.1487) -> (61.073, 46.8313) centre (61.073, 46.99) ccw
  arc A424 (10.4521, 46.8313) -> (10.4521, 47.1487) centre (10.4521, 46.99) ccw
  arc A425 (84.2253, 45.5613) -> (84.2253, 45.8787) centre (84.2253, 45.72) ccw
  arc A426 (81.28, 46.1963) -> (81.28, 46.5138) centre (81.28, 46.3551) ccw
  arc A427 (84.2253, 44.2913) -> (84.2253, 44.6088) centre (84.2253, 44.4501) ccw
  arc A428 (62.7503, 45.5613) -> (62.7503, 45.8787) centre (62.7503, 45.72) ccw
  line L1 (15.353, 46.99) -> (15.7603, 46.99)
  arc A429 (15.988, 46.5138) -> (15.988, 46.1963) centre (15.988, 46.3551) ccw
  arc A430 (0.7747, 45.2437) -> (0.7747, 44.9263) centre (0.7747, 45.085) ccw
  arc A431 (71.8947, 44.9263) -> (71.8947, 45.2437) centre (71.8947, 45.085) ccw
  arc A432 (82.4468, 46.5138) -> (82.4468, 46.1963) centre (82.4468, 46.3551) ccw
  arc A433 (5.9817, 44.2913) -> (5.9817, 44.6088) centre (5.9817, 44.4501) ccw
  arc A434 (0.7747, 45.8787) -> (0.7747, 45.5613) centre (0.7747, 45.72) ccw
  arc A435 (17.258, 45.2437) -> (17.258, 44.9263) centre (17.258, 45.085) ccw
  arc A436 (76.9497, 47.1487) -> (76.9497, 46.8313) centre (76.9497, 46.99) ccw
  arc A437 (81.28, 45.8787) -> (81.28, 45.5613) centre (81.28, 45.72) ccw
  arc A438 (81.28, 46.5138) -> (81.28, 46.1963) centre (81.28, 46.3551) ccw
  arc A439 (80.9625, 48.1013) -> (80.9625, 48.4188) centre (80.9625, 48.2601) ccw
  arc A440 (71.247, 48.1013) -> (71.247, 48.4188) centre (71.247, 48.2601) ccw
  arc A441 (57.6703, 45.5613) -> (57.6703, 45.8787) centre (57.6703, 45.72) ccw
  arc A442 (74.2603, 48.1013) -> (74.2603, 48.4188) centre (74.2603, 48.2601) ccw
  arc A443 (74.4097, 47.1487) -> (74.4097, 46.8313) centre (74.4097, 46.99) ccw
  arc A444 (0.7747, 47.7837) -> (0.7747, 47.4663) centre (0.7747, 47.625) ccw
  arc A445 (59.1697, 45.8787) -> (59.1697, 45.5613) centre (59.1697, 45.72) ccw
  arc A446 (60.438, 47.7837) -> (60.438, 47.4663) centre (60.438, 47.625) ccw
  arc A447 (19.05, 47.7837) -> (19.05, 47.4663) centre (19.05, 47.625) ccw
  arc A448 (15.353, 47.1487) -> (15.353, 46.8313) centre (15.353, 46.99) ccw
  arc A449 (43.702, 46.1963) -> (43.702, 46.5138) centre (43.702, 46.3551) ccw
  arc A450 (42.658, 46.5138) -> (42.658, 46.1963) centre (42.658, 46.3551) ccw
  arc A451 (82.7578, 45.8787) -> (82.7578, 45.5613) centre (82.7578, 45.72) ccw
  arc A452 (0.7747, 47.1487) -> (0.7747, 46.8313) centre (0.7747, 46.99) ccw
  arc A453 (20.8403, 46.8313) -> (20.8403, 47.1487) centre (20.8403, 46.99) ccw
  arc A454 (0.7747, 46.5138) -> (0.7747, 46.1963) centre (0.7747, 46.3551) ccw
  arc A455 (19.05, 47.4663) -> (19.05, 47.7837) centre (19.05, 47.625) ccw
  arc A456 (61.708, 46.5138) -> (61.708, 46.1963) centre (61.708, 46.3551) ccw
  arc A457 (71.247, 46.8313) -> (71.247, 47.1487) centre (71.247, 46.99) ccw
  arc A458 (81.28, 45.5613) -> (81.28, 45.8787) centre (81.28, 45.72) ccw
  arc A459 (16.623, 45.8787) -> (16.623, 45.5613) centre (16.623, 45.72) ccw
  arc A460 (10.4521, 46.1963) -> (10.4521, 46.5138) centre (10.4521, 46.3551) ccw
  arc A461 (22.3397, 47.1487) -> (22.3397, 46.8313) centre (22.3397, 46.99) ccw
  arc A462 (84.2253, 46.1963) -> (84.2253, 46.5138) centre (84.2253, 46.3551) ccw
  arc A463 (61.9379, 45.8787) -> (61.9379, 45.5613) centre (61.9379, 45.72) ccw
  arc A464 (77.9903, 46.8313) -> (77.9903, 47.1487) centre (77.9903, 46.99) ccw
  arc A465 (79.9568, 48.1013) -> (79.9568, 48.4188) centre (79.9568, 48.2601) ccw
  line L2 (4.0005, 48.26) -> (4.6355, 48.26)
  arc A466 (42.023, 45.8787) -> (42.023, 45.5613) centre (42.023, 45.72) ccw
  arc A467 (59.577, 45.5613) -> (59.577, 45.8787) centre (59.577, 45.72) ccw
  arc A468 (59.6465, 48.4188) -> (59.6465, 48.1013) centre (59.6465, 48.2601) ccw
  arc A469 (73.533, 48.4188) -> (73.533, 48.1013) centre (73.533, 48.2601) ccw
  arc A470 (80.3275, 48.4188) -> (80.3275, 48.1013) centre (80.3275, 48.2601) ccw
  arc A471 (75.4503, 46.8313) -> (75.4503, 47.1487) centre (75.4503, 46.99) ccw
  arc A472 (64.2497, 45.8787) -> (64.2497, 45.5613) centre (64.2497, 45.72) ccw
  arc A473 (23.671, 46.1963) -> (23.671, 46.5138) centre (23.671, 46.3551) ccw
  arc A474 (71.4158, 46.1963) -> (71.4158, 46.5138) centre (71.4158, 46.3551) ccw
  arc A475 (4.0005, 48.4188) -> (4.0005, 48.1013) centre (4.0005, 48.2601) ccw
  arc A476 (81.3332, 48.4188) -> (81.3332, 48.1013) centre (81.3332, 48.2601) ccw
  arc A477 (75.5997, 48.4188) -> (75.5997, 48.1013) centre (75.5997, 48.2601) ccw
  arc A478 (34.177, 46.8313) -> (34.177, 47.1487) centre (34.177, 46.99) ccw
  arc A479 (3.6298, 48.1013) -> (3.6298, 48.4188) centre (3.6298, 48.2601) ccw
  arc A480 (19.05, 48.4188) -> (19.05, 48.1013) centre (19.05, 48.2601) ccw
  arc A481 (4.6355, 48.7363) -> (4.6355, 49.0538) centre (4.6355, 48.8951) ccw
  arc A482 (84.2253, 47.4663) -> (84.2253, 47.7837) centre (84.2253, 47.625) ccw
  arc A483 (0.7747, 49.0538) -> (0.7747, 48.7363) centre (0.7747, 48.8951) ccw
  arc A484 (31.3032, 48.4188) -> (31.3032, 48.1013) centre (31.3032, 48.2601) ccw
  arc A485 (34.5821, 47.4663) -> (34.5821, 47.7837) centre (34.5821, 47.625) ccw
  arc A486 (9.6647, 48.1013) -> (9.6647, 48.4188) centre (9.6647, 48.2601) ccw
  arc A487 (31.7935, 48.1013) -> (31.7935, 48.4188) centre (31.7935, 48.2601) ccw
  arc A488 (74.93, 48.4188) -> (74.93, 48.1013) centre (74.93, 48.2601) ccw
  arc A489 (71.247, 47.4663) -> (71.247, 47.7837) centre (71.247, 47.625) ccw
  arc A490 (24.1735, 48.1013) -> (24.1735, 48.4188) centre (24.1735, 48.2601) ccw
  arc A491 (23.3553, 48.4188) -> (23.3553, 48.1013) centre (23.3553, 48.2601) ccw
  arc A492 (27.1168, 48.1013) -> (27.1168, 48.4188) centre (27.1168, 48.2601) ccw
  arc A493 (28.7632, 48.4188) -> (28.7632, 48.1013) centre (28.7632, 48.2601) ccw
  arc A494 (26.6265, 48.4188) -> (26.6265, 48.1013) centre (26.6265, 48.2601) ccw
  arc A495 (34.3335, 48.1013) -> (34.3335, 48.4188) centre (34.3335, 48.2601) ccw
  arc A496 (2.1361, 48.7363) -> (2.1361, 49.0538) centre (2.1361, 48.8951) ccw
  arc A497 (30.48, 48.1013) -> (30.48, 48.4188) centre (30.48, 48.2601) ccw
  arc A498 (84.2253, 48.1013) -> (84.2253, 48.4188) centre (84.2253, 48.2601) ccw
  arc A499 (0.7747, 48.4188) -> (0.7747, 48.1013) centre (0.7747, 48.2601) ccw
  arc A500 (5.0062, 48.4188) -> (5.0062, 48.1013) centre (5.0062, 48.2601) ccw
  arc A501 (27.94, 48.4188) -> (27.94, 48.1013) centre (27.94, 48.2601) ccw
  arc A502 (73.533, 47.7837) -> (73.533, 47.4663) centre (73.533, 47.625) ccw
  arc A503 (59.7335, 48.1013) -> (59.7335, 48.4188) centre (59.7335, 48.2601) ccw
  arc A504 (29.6568, 48.1013) -> (29.6568, 48.4188) centre (29.6568, 48.2601) ccw
  arc A505 (19.05, 48.1013) -> (19.05, 48.4188) centre (19.05, 48.2601) ccw
  arc A506 (62.1865, 48.4188) -> (62.1865, 48.1013) centre (62.1865, 48.2601) ccw
  arc A507 (34.2465, 48.4188) -> (34.2465, 48.1013) centre (34.2465, 48.2601) ccw
  arc A508 (19.05, 50.3237) -> (19.05, 50.0063) centre (19.05, 50.165) ccw
  arc A509 (30.48, 48.4188) -> (30.48, 48.1013) centre (30.48, 48.2601) ccw
  arc A510 (6.4999, 49.0538) -> (6.4999, 48.7363) centre (6.4999, 48.8951) ccw
  arc A511 (27.94, 49.0538) -> (27.94, 48.7363) centre (27.94, 48.8951) ccw
  arc A512 (74.93, 48.1013) -> (74.93, 48.4188) centre (74.93, 48.2601) ccw
  arc A513 (27.94, 48.1013) -> (27.94, 48.4188) centre (27.94, 48.2601) ccw
  arc A514 (4.6355, 48.1013) -> (4.6355, 48.4188) centre (4.6355, 48.2601) ccw
  arc A515 (4.6355, 50.0063) -> (4.6355, 50.3237) centre (4.6355, 50.165) ccw
  arc A516 (9.6647, 49.3713) -> (9.6647, 49.6887) centre (9.6647, 49.53) ccw
  arc A517 (84.2253, 48.7363) -> (84.2253, 49.0538) centre (84.2253, 48.8951) ccw
  arc A518 (19.05, 49.0538) -> (19.05, 48.7363) centre (19.05, 48.8951) ccw
  arc A519 (23.1009, 47.7837) -> (23.1009, 47.4663) centre (23.1009, 47.625) ccw
  arc A520 (77.7787, 49.3713) -> (77.7787, 49.6887) centre (77.7787, 49.53) ccw
  arc A521 (19.05, 48.7363) -> (19.05, 49.0538) centre (19.05, 48.8951) ccw
  arc A522 (0.7747, 49.6887) -> (0.7747, 49.3713) centre (0.7747, 49.53) ccw
  arc A523 (52.1135, 50.6413) -> (52.1135, 50.9588) centre (52.1135, 50.8001) ccw
  arc A524 (30.48, 50.0063) -> (30.48, 50.3237) centre (30.48, 50.165) ccw
  arc A525 (54.6535, 50.6413) -> (54.6535, 50.9588) centre (54.6535, 50.8001) ccw
  arc A526 (4.0005, 49.6887) -> (4.0005, 49.3713) centre (4.0005, 49.53) ccw
  arc A527 (9.6647, 48.7363) -> (9.6647, 49.0538) centre (9.6647, 48.8951) ccw
  arc A528 (31.7935, 50.6413) -> (31.7935, 50.9588) centre (31.7935, 50.8001) ccw
  arc A529 (84.2253, 49.3713) -> (84.2253, 49.6887) centre (84.2253, 49.53) ccw
  arc A530 (82.8269, 49.0538) -> (82.8269, 48.7363) centre (82.8269, 48.8951) ccw
  arc A531 (80.9625, 49.3713) -> (80.9625, 49.6887) centre (80.9625, 49.53) ccw
  arc A532 (4.0005, 50.3237) -> (4.0005, 50.0063) centre (4.0005, 50.165) ccw
  arc A533 (30.48, 49.0538) -> (30.48, 48.7363) centre (30.48, 48.8951) ccw
  arc A534 (78.4631, 48.7363) -> (78.4631, 49.0538) centre (78.4631, 48.8951) ccw
  arc A535 (27.94, 48.7363) -> (27.94, 49.0538) centre (27.94, 48.8951) ccw
  arc A536 (70.7644, 48.7363) -> (70.7644, 49.0538) centre (70.7644, 48.8951) ccw
  arc A537 (80.3275, 49.6887) -> (80.3275, 49.3713) centre (80.3275, 49.53) ccw
  arc A538 (80.3275, 49.0538) -> (80.3275, 48.7363) centre (80.3275, 48.8951) ccw
  arc A539 (70.7644, 49.3713) -> (70.7644, 49.6887) centre (70.7644, 49.53) ccw
  arc A540 (74.93, 49.0538) -> (74.93, 48.7363) centre (74.93, 48.8951) ccw
  arc A541 (27.94, 50.3237) -> (27.94, 50.0063) centre (27.94, 50.165) ccw
  arc A542 (74.93, 48.7363) -> (74.93, 49.0538) centre (74.93, 48.8951) ccw
  arc A543 (4.0005, 49.0538) -> (4.0005, 48.7363) centre (4.0005, 48.8951) ccw
  arc A544 (0.7747, 50.3237) -> (0.7747, 50.0063) centre (0.7747, 50.165) ccw
  arc A545 (80.9625, 48.7363) -> (80.9625, 49.0538) centre (80.9625, 48.8951) ccw
  arc A546 (62.6077, 49.0538) -> (62.6077, 48.7363) centre (62.6077, 48.8951) ccw
  arc A547 (27.94, 50.0063) -> (27.94, 50.3237) centre (27.94, 50.165) ccw
  arc A548 (7.1843, 49.6887) -> (7.1843, 49.3713) centre (7.1843, 49.53) ccw
  arc A549 (1.4517, 49.3713) -> (1.4517, 49.6887) centre (1.4517, 49.53) ccw
  arc A550 (74.93, 49.6887) -> (74.93, 49.3713) centre (74.93, 49.53) ccw
  arc A551 (19.05, 50.0063) -> (19.05, 50.3237) centre (19.05, 50.165) ccw
  arc A552 (62.7253, 49.6887) -> (62.7253, 49.3713) centre (62.7253, 49.53) ccw
  arc A553 (30.48, 49.3713) -> (30.48, 49.6887) centre (30.48, 49.53) ccw
  arc A554 (76.2347, 49.0538) -> (76.2347, 48.7363) centre (76.2347, 48.8951) ccw
  arc A555 (83.5113, 49.6887) -> (83.5113, 49.3713) centre (83.5113, 49.53) ccw
  arc A556 (7.6157, 50.3237) -> (7.6157, 50.0063) centre (7.6157, 50.165) ccw
  arc A557 (4.6355, 49.3713) -> (4.6355, 49.6887) centre (4.6355, 49.53) ccw
  arc A558 (1.0202, 50.0063) -> (1.0202, 50.3237) centre (1.0202, 50.165) ccw
  arc A559 (30.48, 48.7363) -> (30.48, 49.0538) centre (30.48, 48.8951) ccw
  arc A560 (9.6647, 50.0063) -> (9.6647, 50.3237) centre (9.6647, 50.165) ccw
  line L3 (27.94, 49.53) -> (30.48, 49.53)
  arc A561 (41.9535, 50.6413) -> (41.9535, 50.9588) centre (41.9535, 50.8001) ccw
  arc A562 (49.4865, 50.9588) -> (49.4865, 50.6413) centre (49.4865, 50.8001) ccw
  arc A563 (30.48, 50.3237) -> (30.48, 50.0063) centre (30.48, 50.165) ccw
  arc A564 (52.0265, 50.9588) -> (52.0265, 50.6413) centre (52.0265, 50.8001) ccw
  arc A565 (27.94, 49.6887) -> (27.94, 49.3713) centre (27.94, 49.53) ccw
  arc A566 (70.7644, 50.0063) -> (70.7644, 50.3237) centre (70.7644, 50.165) ccw
  arc A567 (39.3265, 50.9588) -> (39.3265, 50.6413) centre (39.3265, 50.8001) ccw
  arc A568 (84.2253, 50.0063) -> (84.2253, 50.3237) centre (84.2253, 50.165) ccw
  arc A569 (54.5665, 50.9588) -> (54.5665, 50.6413) centre (54.5665, 50.8001) ccw
  arc A570 (80.3275, 50.3237) -> (80.3275, 50.0063) centre (80.3275, 50.165) ccw
  arc A571 (36.8735, 50.6413) -> (36.8735, 50.9588) centre (36.8735, 50.8001) ccw
  arc A572 (19.05, 50.6413) -> (19.05, 50.9588) centre (19.05, 50.8001) ccw
  arc A573 (39.4135, 50.6413) -> (39.4135, 50.9588) centre (39.4135, 50.8001) ccw
  arc A574 (47.0335, 50.6413) -> (47.0335, 50.9588) centre (47.0335, 50.8001) ccw
  arc A575 (23.3553, 50.9588) -> (23.3553, 50.6413) centre (23.3553, 50.8001) ccw
  arc A576 (49.5735, 50.6413) -> (49.5735, 50.9588) centre (49.5735, 50.8001) ccw
  arc A577 (44.4935, 50.6413) -> (44.4935, 50.9588) centre (44.4935, 50.8001) ccw
  arc A578 (30.48, 50.6413) -> (30.48, 50.9588) centre (30.48, 50.8001) ccw
  arc A579 (29.6568, 50.6413) -> (29.6568, 50.9588) centre (29.6568, 50.8001) ccw
  arc A580 (27.94, 50.9588) -> (27.94, 50.6413) centre (27.94, 50.8001) ccw
  arc A581 (15.7603, 51.9113) -> (15.7603, 52.2287) centre (15.7603, 52.07) ccw
  arc A582 (30.48, 50.9588) -> (30.48, 50.6413) centre (30.48, 50.8001) ccw
  arc A583 (36.7865, 50.9588) -> (36.7865, 50.6413) centre (36.7865, 50.8001) ccw
  arc A584 (4.6355, 50.6413) -> (4.6355, 50.9588) centre (4.6355, 50.8001) ccw
  arc A585 (26.6265, 50.9588) -> (26.6265, 50.6413) centre (26.6265, 50.8001) ccw
  arc A586 (9.6647, 50.6413) -> (9.6647, 50.9588) centre (9.6647, 50.8001) ccw
  arc A587 (31.3032, 50.9588) -> (31.3032, 50.6413) centre (31.3032, 50.8001) ccw
  arc A588 (4.0005, 50.9588) -> (4.0005, 50.6413) centre (4.0005, 50.8001) ccw
  arc A589 (77.4969, 53.8163) -> (77.4969, 54.1337) centre (77.4969, 53.975) ccw
  arc A590 (74.93, 50.3237) -> (74.93, 50.0063) centre (74.93, 50.165) ccw
  arc A591 (7.4661, 54.1337) -> (7.4661, 53.8163) centre (7.4661, 53.975) ccw
  arc A592 (4.6355, 52.2287) -> (4.6355, 51.9113) centre (4.6355, 52.07) ccw
  arc A593 (80.9625, 50.0063) -> (80.9625, 50.3237) centre (80.9625, 50.165) ccw
  arc A594 (44.4065, 50.9588) -> (44.4065, 50.6413) centre (44.4065, 50.8001) ccw
  arc A595 (83.9427, 50.3237) -> (83.9427, 50.0063) centre (83.9427, 50.165) ccw
  arc A596 (71.3611, 50.6413) -> (71.3611, 50.9588) centre (71.3611, 50.8001) ccw
  arc A597 (46.9465, 50.9588) -> (46.9465, 50.6413) centre (46.9465, 50.8001) ccw
  arc A598 (34.3335, 50.6413) -> (34.3335, 50.9588) centre (34.3335, 50.8001) ccw
  arc A599 (7.7945, 53.4988) -> (7.7945, 53.1813) centre (7.7945, 53.3401) ccw
  arc A600 (78.0136, 54.4513) -> (78.0136, 54.7687) centre (78.0136, 54.61) ccw
  arc A601 (7.8864, 50.9588) -> (7.8864, 50.6413) centre (7.8864, 50.8001) ccw
  arc A602 (77.3472, 50.0063) -> (77.3472, 50.3237) centre (77.3472, 50.165) ccw
  arc A603 (34.2465, 50.9588) -> (34.2465, 50.6413) centre (34.2465, 50.8001) ccw
  arc A604 (28.7632, 50.9588) -> (28.7632, 50.6413) centre (28.7632, 50.8001) ccw
  arc A605 (62.6077, 50.3237) -> (62.6077, 50.0063) centre (62.6077, 50.165) ccw
  arc A606 (27.1168, 50.6413) -> (27.1168, 50.9588) centre (27.1168, 50.8001) ccw
  arc A607 (74.93, 50.0063) -> (74.93, 50.3237) centre (74.93, 50.165) ccw
  arc A608 (76.2347, 50.3237) -> (76.2347, 50.0063) centre (76.2347, 50.165) ccw
  arc A609 (41.8665, 50.9588) -> (41.8665, 50.6413) centre (41.8665, 50.8001) ccw
  arc A610 (27.94, 50.6413) -> (27.94, 50.9588) centre (27.94, 50.8001) ccw
  arc A611 (24.1735, 50.6413) -> (24.1735, 50.9588) centre (24.1735, 50.8001) ccw
  arc A612 (19.05, 50.9588) -> (19.05, 50.6413) centre (19.05, 50.8001) ccw
  arc A613 (74.2603, 50.6413) -> (74.2603, 50.9588) centre (74.2603, 50.8001) ccw
  arc A614 (77.1685, 53.1813) -> (77.1685, 53.4988) centre (77.1685, 53.3401) ccw
  arc A615 (12.1797, 52.2287) -> (12.1797, 51.9113) centre (12.1797, 52.07) ccw
  arc A616 (19.05, 51.5938) -> (19.05, 51.2763) centre (19.05, 51.4351) ccw
  arc A617 (6.9493, 54.7687) -> (6.9493, 54.4513) centre (6.9493, 54.61) ccw
  arc A618 (84.2134, 50.9588) -> (84.2134, 50.6413) centre (84.2134, 50.8001) ccw
  arc A619 (74.93, 50.6413) -> (74.93, 50.9588) centre (74.93, 50.8001) ccw
  arc A620 (9.9191, 51.2763) -> (9.9191, 51.5938) centre (9.9191, 51.4351) ccw
  arc A621 (76.9304, 51.2763) -> (76.9304, 51.5938) centre (76.9304, 51.4351) ccw
  arc A622 (20.8403, 51.9113) -> (20.8403, 52.2287) centre (20.8403, 52.07) ccw
  arc A623 (80.9625, 51.2763) -> (80.9625, 51.5938) centre (80.9625, 51.4351) ccw
  arc A624 (10.16, 41.8338) -> (10.16, 41.9862) centre (10.16, 41.91) ccw
  line L4 (73.4189, 50.8) -> (74.2603, 50.8)
  arc A625 (73.4189, 50.9588) -> (73.4189, 50.6413) centre (73.4189, 50.8001) ccw